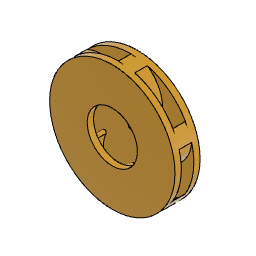
_IMPELLER FINAL.05714027-a7b8-42e8-8b00-f8052b93d887_LV3 (Autodesk Fusion 360 design; units mm, degrees)
Autodesk Fusion 360 part; units mm, degrees
sketch "Sketch1" plane through (0, 0, 0) normal (0, 1, 0) x (1, 0, 0)
  circle A0 centre (0, 0) radius 50
  circle A1 centre (0, 0) radius 25 construction
  arc A2 (0, -50) -> (20, -15) centre (-2.8415, -25.162) ccw
  arc A3 (12.9263, -48.3002) -> (22.741, -13.7806) centre (-2.8415, -25.162) ccw
  arc A4 (22.741, -13.7806) -> (20, -15) centre (21.3705, -14.3903) ccw
  line L0 (0, -1.75) -> (0, -22.5)
  arc A5 (23.3048, 12.804) -> (22.9904, 9.8205) centre (23.1476, 11.3122) ccw
  arc A6 (43.3013, -25) -> (22.9904, 9.8205) centre (20.3702, -15.0418) ccw
  arc A7 (48.2924, -12.9556) -> (23.3048, 12.804) centre (20.3702, -15.0418) ccw
  arc A8 (0.5638, 26.5845) -> (2.9904, 24.8205) centre (1.7771, 25.7025) ccw
  arc A9 (43.3013, 25) -> (2.9904, 24.8205) centre (23.2117, 10.1202) ccw
  arc A10 (35.3661, 35.3446) -> (0.5638, 26.5845) centre (23.2117, 10.1202) ccw
  arc A11 (-22.741, 13.7806) -> (-20, 15) centre (-21.3705, 14.3903) ccw
  arc A12 (0, 50) -> (-20, 15) centre (2.8415, 25.162) ccw
  arc A13 (-12.9263, 48.3002) -> (-22.741, 13.7806) centre (2.8415, 25.162) ccw
  arc A14 (-23.3048, -12.804) -> (-22.9904, -9.8205) centre (-23.1476, -11.3122) ccw
  arc A15 (-43.3013, 25) -> (-22.9904, -9.8205) centre (-20.3702, 15.0418) ccw
  arc A16 (-48.2924, 12.9556) -> (-23.3048, -12.804) centre (-20.3702, 15.0418) ccw
  arc A17 (-0.5638, -26.5845) -> (-2.9904, -24.8205) centre (-1.7771, -25.7025) ccw
  arc A18 (-43.3013, -25) -> (-2.9904, -24.8205) centre (-23.2117, -10.1202) ccw
  arc A19 (-35.3661, -35.3446) -> (-0.5638, -26.5845) centre (-23.2117, -10.1202) ccw
  dimension "d1" = 100
  dimension "d2" = 50
  dimension "d6" = 1.5
  dimension "d7" = 25
  dimension "d9" = 360
  constraint coincident A0.centre A1.centre
  constraint concentric A0 A1
  constraint coincident A0 A2.start
  constraint coincident A1 A2.end
  constraint coincident A2.start L0
  constraint concentric A2 A3
  constraint coincident A0 A3.start
  constraint tangent A2 A4
  constraint tangent A3 A4
  measures "d1" diameter of A0
  measures "d2" diameter of A1
  measures "d6" radius of A4
  measures "d7" radius of A2
extrude "Extrude1" add sketch "Sketch1" against normal blind 10 contours A0 A8 A9 A10 | A0 A5 A6 A7 | A0 A11 A12 A13 | A0 A2 A3 A4 | A0 A14 A15 A16 | A0 A17 A18 A19 makes body 1 at (4.4955, -6.6667, -26.6944) makes body 2 at (-20.1028, -6.6667, 34.9262) makes body 3 at (-20.1955, -6.6667, -34.8726) makes body 4 at (43.3198, -6.6667, 5.1264) makes body 5 at (20.4621, -6.6667, 16.1098) makes body 6 at (-25.3658, -6.6667, 9.454)
sketch "Sketch2" plane through (0, 0, 0) normal (0, 1, 0) x (1, 0, 0)
  circle A0 centre (0, 0) radius 50
  constraint coincident A0.centre origin
extrude "Extrude2" add sketch "Sketch2" along normal blind 5 bodies 1 2 3 4 5 6
ref_plane "WorkPlane1" through (0, -10, 0) normal (0, 1, 0) x (0, 0, 1)
sketch "Sketch3" plane through (0, -10, 0) normal (0, 1, 0) x (1, 0, 0)
  circle A0 centre (0, 0) radius 50
  dimension "d15" = 100
  constraint coincident A0.centre origin
  measures "d15" diameter of A0
extrude "Extrude3" add sketch "Sketch3" against normal blind 5 separate body makes body 7
combine "Combine1" operation add target body 7 tool bodies 1
hole "Hole1" at (0, -15, 0) direction (0, 1, 0) diameter 40 depth 15 tip angle 180 bodies 7
sketch "Sketch4" plane through (0, 0, 0) normal (0, 1, 0) x (1, 0, 0)
  circle A0 centre (0, 0) radius 5
  circle A1 centre (0, 0) radius 2.5
  dimension "d21" = 10
  dimension "d22" = 5
  constraint coincident A0.centre A1.centre
  measures "d21" diameter of A0
  measures "d22" diameter of A1
hole "Hole2" at (-0.0204, 0, 0.0738) direction (0, 1, 0) diameter 5 depth 50 tip angle 180 bodies 7
extrude "Extrude5" add sketch "Sketch4" along normal blind 10 bodies 7
named bodies: "Impeller"
